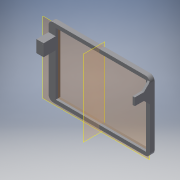
# Autodesk Inventor part: 07_Omnivision_wellplate_traystage
Saved by Autodesk Inventor 2019.4 (Build 234330000, 330)
## iProperties
Created: 2021-09-28
Part Number: 07_Omnivision_wellplate_traystage
Material: Generic
Document SubType Name: Modeling
Designer: diederichbenedict
Density: 1 g/cm^3
Appearance: Default
Author: diederichbenedict
Autodesk Inventor part; units mm, degrees
ref_plane "YZ Plane" through (0, 0, 0) normal (1, 0, 0) x (0, 1, 0)
ref_plane "XZ Plane" through (0, 0, 0) normal (0, 1, 0) x (-1, 0, 0)
ref_plane "XY Plane" through (0, 0, 0) normal (0, 0, 1) x (1, 0, 0)
ref_plane "Work Plane1" through (-7.109, -3.9363, 0) normal (0, 0, 1) x (1, 0, 0)
sketch "Sketch1" plane through (-7.109, -3.9363, 0) normal (0, 0, 1) x (1, 0, 0)
  line L0 (71.054, 43.7363) -> (71.054, -35.8637) construction
  arc A0 (71.054, 43.7363) -> (68.054, 46.7363) centre (68.054, 43.7363) ccw construction
  line L1 (-53.836, 46.7363) -> (68.054, 46.7363) construction
  arc A1 (-53.836, 46.7363) -> (-56.836, 43.7363) centre (-53.836, 43.7363) ccw construction
  line L2 (-56.836, -35.8637) -> (-56.836, 43.7363) construction
  arc A2 (-56.836, -35.8637) -> (-53.836, -38.8637) centre (-53.836, -35.8637) ccw construction
  line L3 (68.054, -38.8637) -> (-53.836, -38.8637) construction
  arc A3 (68.054, -38.8637) -> (71.054, -35.8637) centre (68.054, -35.8637) ccw construction
  line L4 (-56.516, -35.5437) -> (-56.516, 43.4163) construction
  arc A4 (-53.516, 46.4163) -> (-56.516, 43.4163) centre (-53.516, 43.4163) ccw construction
  line L5 (-53.516, 46.4163) -> (67.734, 46.4163) construction
  arc A5 (70.734, 43.4163) -> (67.734, 46.4163) centre (67.734, 43.4163) ccw construction
  line L6 (70.734, 43.4163) -> (70.734, -35.5437) construction
  arc A6 (67.734, -38.5437) -> (70.734, -35.5437) centre (67.734, -35.5437) ccw construction
  line L7 (67.734, -38.5437) -> (-53.516, -38.5437) construction
  arc A7 (-56.516, -35.5437) -> (-53.516, -38.5437) centre (-53.516, -35.5437) ccw construction
  arc A8 (75.054, 43.7363) -> (68.054, 50.7363) centre (68.054, 43.7363) ccw
  line L8 (75.054, 43.7363) -> (75.054, -35.8637)
  arc A9 (68.054, -42.8637) -> (75.054, -35.8637) centre (68.054, -35.8637) ccw
  line L9 (68.054, -42.8637) -> (-53.836, -42.8637)
  arc A10 (-60.836, -35.8637) -> (-53.836, -42.8637) centre (-53.836, -35.8637) ccw
  line L10 (-60.836, -35.8637) -> (-60.836, 43.7363)
  arc A11 (-53.836, 50.7363) -> (-60.836, 43.7363) centre (-53.836, 43.7363) ccw
  line L11 (-53.836, 50.7363) -> (68.054, 50.7363)
  circle A12 centre (53.6173, 21.8363) radius 4 construction
  circle A13 centre (53.6173, 3.8363) radius 4 construction
  circle A14 centre (53.6173, -14.1637) radius 4 construction
  circle A15 centre (35.6173, 21.8363) radius 4 construction
  circle A16 centre (35.6173, 3.8363) radius 4 construction
  circle A17 centre (35.6173, -14.1637) radius 4 construction
  circle A18 centre (17.6173, 21.8363) radius 4 construction
  circle A19 centre (17.6173, 3.8363) radius 4 construction
  circle A20 centre (17.6173, -14.1637) radius 4 construction
  circle A21 centre (-0.3827, 21.8363) radius 4 construction
  circle A22 centre (-0.3827, 3.8363) radius 4 construction
  circle A23 centre (-0.3827, -14.1637) radius 4 construction
  circle A24 centre (-18.3827, 21.8363) radius 4 construction
  circle A25 centre (-18.3827, 3.8363) radius 4 construction
  circle A26 centre (-18.3827, -14.1637) radius 4 construction
  circle A27 centre (-36.3827, 21.8363) radius 4 construction
  circle A28 centre (-36.3827, 3.8363) radius 4 construction
  circle A29 centre (-36.3827, -14.1637) radius 4 construction
  circle A30 centre (-36.3827, 30.7863) radius 4.375 construction
  circle A31 centre (-18.3827, 30.7863) radius 4.375 construction
  circle A32 centre (-0.3827, 30.7863) radius 4.375 construction
  circle A33 centre (17.6173, 30.7863) radius 4.375 construction
  circle A34 centre (35.6173, 30.7863) radius 4.375 construction
  circle A35 centre (53.6173, 30.7863) radius 4.375 construction
  circle A36 centre (-36.3827, 12.7863) radius 4.375 construction
  circle A37 centre (-18.3827, 12.7863) radius 4.375 construction
  circle A38 centre (-0.3827, 12.7863) radius 4.375 construction
  circle A39 centre (17.6173, 12.7863) radius 4.375 construction
  circle A40 centre (35.6173, 12.7863) radius 4.375 construction
  circle A41 centre (53.6173, 12.7863) radius 4.375 construction
  circle A42 centre (-36.3827, -5.2137) radius 4.375 construction
  circle A43 centre (-18.3827, -5.2137) radius 4.375 construction
  circle A44 centre (-0.3827, -5.2137) radius 4.375 construction
  circle A45 centre (17.6173, -5.2137) radius 4.375 construction
  circle A46 centre (35.6173, -5.2137) radius 4.375 construction
  circle A47 centre (53.6173, -5.2137) radius 4.375 construction
  circle A48 centre (-36.3827, -23.2137) radius 4.375 construction
  circle A49 centre (-18.3827, -23.2137) radius 4.375 construction
  circle A50 centre (-0.3827, -23.2137) radius 4.375 construction
  circle A51 centre (17.6173, -23.2137) radius 4.375 construction
  circle A52 centre (35.6173, -23.2137) radius 4.375 construction
  circle A53 centre (53.6173, -23.2137) radius 4.375 construction
  arc A54 (57.7361, 42.9363) -> (61.1439, 37.9635) centre (61.609, 41.9363) ccw construction
  line L12 (-39.518, 42.9363) -> (57.7361, 42.9363) construction
  arc A55 (-42.9259, 37.9635) -> (-39.518, 42.9363) centre (-43.391, 41.9363) ccw construction
  arc A56 (-48.391, 33.7282) -> (-42.9259, 37.9635) centre (-46.891, 37.4363) ccw construction
  line L13 (-48.391, -25.8556) -> (-48.391, 33.7282) construction
  arc A57 (-42.9259, -30.0908) -> (-48.391, -25.8556) centre (-46.891, -29.5637) ccw construction
  arc A58 (-39.518, -35.0637) -> (-42.9259, -30.0908) centre (-43.391, -34.0637) ccw construction
  line L14 (57.7361, -35.0637) -> (-39.518, -35.0637) construction
  arc A59 (61.1439, -30.0908) -> (57.7361, -35.0637) centre (61.609, -34.0637) ccw construction
  arc A60 (66.609, -25.8556) -> (61.1439, -30.0908) centre (65.109, -29.5637) ccw construction
  line L15 (66.609, 33.7282) -> (66.609, -25.8556) construction
  arc A61 (61.1439, 37.9635) -> (66.609, 33.7282) centre (65.109, 37.4363) ccw construction
  arc A62 (67.609, -27.9054) -> (62.6207, -31.2394) centre (65.109, -29.5637) ccw construction
  arc A63 (62.6207, -31.2394) -> (59.373, -36.0637) centre (61.609, -34.0637) ccw construction
  line L16 (59.373, -36.0637) -> (-41.1549, -36.0637) construction
  arc A64 (-41.1549, -36.0637) -> (-44.4026, -31.2394) centre (-43.391, -34.0637) ccw construction
  arc A65 (-44.4026, -31.2394) -> (-49.391, -27.9054) centre (-46.891, -29.5637) ccw construction
  line L17 (-49.391, -27.9054) -> (-49.391, 35.778) construction
  arc A66 (-49.391, 35.778) -> (-44.4026, 39.112) centre (-46.891, 37.4363) ccw construction
  arc A67 (-44.4026, 39.112) -> (-41.1549, 43.9363) centre (-43.391, 41.9363) ccw construction
  line L18 (-41.1549, 43.9363) -> (59.373, 43.9363) construction
  arc A68 (59.373, 43.9363) -> (62.6207, 39.112) centre (61.609, 41.9363) ccw construction
  arc A69 (62.6207, 39.112) -> (67.609, 35.778) centre (65.109, 37.4363) ccw construction
  line L19 (67.609, 35.778) -> (67.609, -27.9054) construction
  line L20 (69.609, 45.9363) -> (-51.391, 45.9363)
  line L21 (-51.391, 45.9363) -> (-51.391, -38.0637)
  line L22 (-51.391, -38.0637) -> (69.609, -38.0637)
  line L23 (69.609, -38.0637) -> (69.609, 45.9363)
  point P0 (7.109, 3.9363)
  dimension "d0" = 4
  dimension "d1" = 1
  dimension "d10" = 2
  dimension "d11" = 2
  dimension "d12" = 2
  dimension "d13" = 2
  constraints: 24 end point, 24 point on circle, 12 centre point, 2 parallel, 1 horizontal, 1 perpendicular, 18 other
  measures "d0" radial gap between concentric circles of A0 A8
  measures "d1" distance between parallel lines of L19 L15
  measures "d10" distance between parallel lines of L22 L16
  measures "d11" distance between parallel lines of L19 L23
  measures "d12" distance between parallel lines of L20 L18
  measures "d13" distance between parallel lines of L17 L21
extrude "Extrusion1" add sketch "Sketch1" along normal blind 3
sketch "Sketch2" plane through (-7.109, -3.9363, 0) normal (0, 0, -1) x (-1, 0, 0)
  line L0 (-71.054, 43.7363) -> (-71.054, -35.8637) construction
  arc A0 (-68.054, 46.7363) -> (-71.054, 43.7363) centre (-68.054, 43.7363) ccw construction
  line L1 (53.836, 46.7363) -> (-68.054, 46.7363) construction
  arc A1 (56.836, 43.7363) -> (53.836, 46.7363) centre (53.836, 43.7363) ccw construction
  line L2 (56.836, -35.8637) -> (56.836, 43.7363) construction
  arc A2 (53.836, -38.8637) -> (56.836, -35.8637) centre (53.836, -35.8637) ccw construction
  line L3 (-68.054, -38.8637) -> (53.836, -38.8637) construction
  arc A3 (-71.054, -35.8637) -> (-68.054, -38.8637) centre (-68.054, -35.8637) ccw construction
  line L4 (56.516, -35.5437) -> (56.516, 43.4163) construction
  arc A4 (56.516, 43.4163) -> (53.516, 46.4163) centre (53.516, 43.4163) ccw construction
  line L5 (53.516, 46.4163) -> (-67.734, 46.4163) construction
  arc A5 (-67.734, 46.4163) -> (-70.734, 43.4163) centre (-67.734, 43.4163) ccw construction
  line L6 (-70.734, 43.4163) -> (-70.734, -35.5437) construction
  arc A6 (-70.734, -35.5437) -> (-67.734, -38.5437) centre (-67.734, -35.5437) ccw construction
  line L7 (-67.734, -38.5437) -> (53.516, -38.5437) construction
  arc A7 (53.516, -38.5437) -> (56.516, -35.5437) centre (53.516, -35.5437) ccw construction
  arc A8 (-68.054, 47.2363) -> (-71.554, 43.7363) centre (-68.054, 43.7363) ccw
  line L8 (-71.554, 43.7363) -> (-71.554, -35.8637)
  arc A9 (-71.554, -35.8637) -> (-68.054, -39.3637) centre (-68.054, -35.8637) ccw
  line L9 (-68.054, -39.3637) -> (53.836, -39.3637)
  arc A10 (53.836, -39.3637) -> (57.336, -35.8637) centre (53.836, -35.8637) ccw
  line L10 (57.336, -35.8637) -> (57.336, 43.7363)
  arc A11 (57.336, 43.7363) -> (53.836, 47.2363) centre (53.836, 43.7363) ccw
  line L11 (53.836, 47.2363) -> (-68.054, 47.2363)
  arc A12 (56.216, 43.4163) -> (53.516, 46.1163) centre (53.516, 43.4163) ccw
  line L12 (56.216, 43.4163) -> (56.216, -35.5437)
  arc A13 (53.516, -38.2437) -> (56.216, -35.5437) centre (53.516, -35.5437) ccw
  line L13 (53.516, -38.2437) -> (-67.734, -38.2437)
  arc A14 (-70.434, -35.5437) -> (-67.734, -38.2437) centre (-67.734, -35.5437) ccw
  line L14 (-70.434, -35.5437) -> (-70.434, 43.4163)
  arc A15 (-67.734, 46.1163) -> (-70.434, 43.4163) centre (-67.734, 43.4163) ccw
  line L15 (-67.734, 46.1163) -> (53.516, 46.1163)
  line L16 (-69.609, 45.9363) -> (-69.609, -38.0637) projected
  line L17 (-69.609, -38.0637) -> (51.391, -38.0637) projected
  line L18 (51.391, -38.0637) -> (51.391, 45.9363) projected
  line L19 (51.391, 45.9363) -> (-69.609, 45.9363) projected
  arc A16 (-68.054, 50.7363) -> (-75.054, 43.7363) centre (-68.054, 43.7363) ccw projected
  line L20 (-68.054, 50.7363) -> (53.836, 50.7363) projected
  arc A17 (60.836, 43.7363) -> (53.836, 50.7363) centre (53.836, 43.7363) ccw projected
  line L21 (60.836, 43.7363) -> (60.836, -35.8637) projected
  arc A18 (53.836, -42.8637) -> (60.836, -35.8637) centre (53.836, -35.8637) ccw projected
  line L22 (53.836, -42.8637) -> (-68.054, -42.8637) projected
  arc A19 (-75.054, -35.8637) -> (-68.054, -42.8637) centre (-68.054, -35.8637) ccw projected
  line L23 (-75.054, -35.8637) -> (-75.054, 43.7363) projected
  point P0 (-7.109, 3.9363)
  dimension "d4" = 0.5
  dimension "d5" = 0.3
  constraints: 16 end point, 16 point on circle, 8 centre point, 14 other
  measures "d4" distance between parallel lines of L1 L11
  measures "d5" radial gap between concentric circles of A4 A12
extrude "Extrusion2" add sketch "Sketch2" along normal blind 3 contours L12 A13 L13 A14 L17 L18 L19 A15 L15 A12 | L16 A14 L14 A15 | L20 A17 L21 A18 L22 A19 L23 A16
sketch "Sketch3" plane through (-7.109, -3.9363, 3) normal (0, 0, 1) x (1, 0, 0)
  line L0 (69.609, 45.9363) -> (69.609, -38.0637) projected
  line L1 (69.609, -38.0637) -> (-51.391, -38.0637) projected
  line L2 (-51.391, -38.0637) -> (-51.391, 45.9363) projected
  line L3 (-51.391, 45.9363) -> (69.609, 45.9363) projected
  arc A0 (75.054, 43.7363) -> (68.054, 50.7363) centre (68.054, 43.7363) ccw projected
  line L4 (68.054, 50.7363) -> (-53.836, 50.7363) projected
  arc A1 (-53.836, 50.7363) -> (-60.836, 43.7363) centre (-53.836, 43.7363) ccw projected
  line L5 (-60.836, 43.7363) -> (-60.836, -35.8637) projected
  arc A2 (-60.836, -35.8637) -> (-53.836, -42.8637) centre (-53.836, -35.8637) ccw projected
  line L6 (-53.836, -42.8637) -> (68.054, -42.8637) projected
  arc A3 (68.054, -42.8637) -> (75.054, -35.8637) centre (68.054, -35.8637) ccw projected
  line L7 (75.054, -35.8637) -> (75.054, 43.7363) projected
  line L8 (75.054, 25.8105) -> (71.9538, 25.8105)
  line L9 (70.434, 43.4163) -> (70.434, -35.5437) projected
  arc A4 (75.054, 43.7363) -> (68.054, 50.7363) centre (68.054, 43.7363) ccw projected
  line L10 (75.054, 28.7363) -> (72.054, 28.7363)
  line L11 (72.054, 28.7363) -> (72.054, 38.7363)
  line L12 (72.054, 38.7363) -> (75.054, 38.7363)
  line L13 (75.054, 38.7363) -> (75.054, 28.7363)
  point P0 (7.109, 3.9363)
  point P1 (71.7253, 49.6963)
  dimension "d14" = 3
  dimension "d15" = 10
  dimension "d16" = 12
  constraints: 10 end point, 2 parallel, 2 perpendicular, 2 point on line, 1 horizontal, 1 point on circle
  measures "d14" distance of L11.end L12.end
  measures "d15" distance of L10.end L11.end
  measures "d16" distance between parallel lines of L12 L4
extrude "Extrusion3" add sketch "Sketch3" along normal blind 20 contours L7 L10 L11 L12
chamfer "Chamfer1" distance 8 angle 45 2 edges at (66.445, 24.8, 3) (66.445, 34.8, 3)
ref_plane "Work Plane2" through (0, -39.8, -3) normal (1, 0, 0) x (0, 0, -1)
sketch "Sketch4" plane through (-7.109, -3.9363, 3) normal (0, 0, 1) x (1, 0, 0)
  line L0 (74.3786, 46.7363) -> (72.054, 46.7363) projected
  arc A0 (74.3786, 46.7363) -> (68.054, 50.7363) centre (68.054, 43.7363) ccw projected
  line L1 (68.054, 50.7363) -> (-53.836, 50.7363) projected
  arc A1 (-53.836, 50.7363) -> (-60.836, 43.7363) centre (-53.836, 43.7363) ccw projected
  line L2 (-60.836, 43.7363) -> (-60.836, -35.8637) projected
  arc A2 (-60.836, -35.8637) -> (-53.836, -42.8637) centre (-53.836, -35.8637) ccw projected
  line L3 (-53.836, -42.8637) -> (68.054, -42.8637) projected
  arc A3 (68.054, -42.8637) -> (75.054, -35.8637) centre (68.054, -35.8637) ccw projected
  line L4 (75.054, -35.8637) -> (75.054, 20.7363) projected
  line L5 (72.054, 20.7363) -> (75.054, 20.7363) projected
  line L6 (72.054, 20.7363) -> (72.054, 46.7363) projected
  line L7 (69.609, 45.9363) -> (69.609, -38.0637) projected
  line L8 (69.609, -38.0637) -> (-51.391, -38.0637) projected
  line L9 (-51.391, -38.0637) -> (-51.391, 45.9363) projected
  line L10 (-51.391, 45.9363) -> (69.609, 45.9363) projected
  circle A4 centre (-51.891, 33.9363) radius 0.5 projected
  line L11 (-49.391, 30.9363) -> (-49.391, 36.9363) projected
  line L12 (-49.391, 36.9363) -> (-54.391, 36.9363) projected
  line L13 (-54.391, 30.9363) -> (-54.391, 36.9363) projected
  line L14 (-49.391, 30.9363) -> (-54.391, 30.9363) projected
  line L15 (-51.391, -38.0637) -> (-51.391, 45.9363) projected
  line L16 (-60.836, -35.8637) -> (-60.836, 43.7363) projected
  line L17 (-51.391, 35.4207) -> (-60.836, 35.4207)
  line L18 (-60.836, 35.4207) -> (-60.836, 19.4207)
  line L19 (-60.836, 19.4207) -> (-51.391, 19.4207)
  line L20 (-51.391, 19.4207) -> (-51.391, 35.4207)
  point P0 (7.109, 3.9363)
  dimension "d20" = 16
  constraints: 8 end point, 2 parallel, 2 point on line, 1 horizontal, 1 perpendicular
  measures "d20" distance of L18.end L17.end
extrude "Extrusion4" add sketch "Sketch4" along normal blind 16 contours L17 L13 L14 L9 L19 L2 | L17 L9 L14 L13
equation "\"d10\" = d11"
equation "\"d12\" = d11"
equation "\"d13\" = d11"
body "Solid1"
